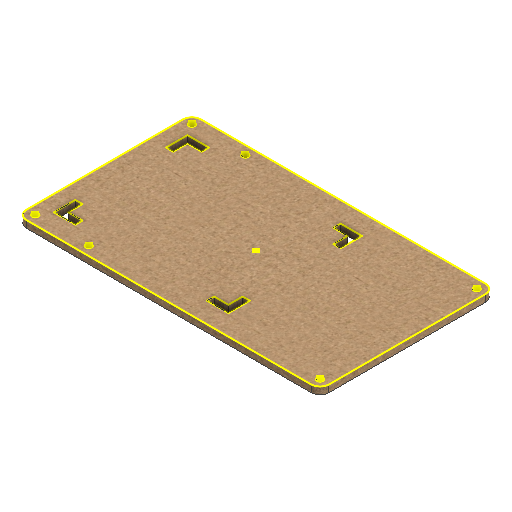
# Autodesk Inventor part: upper_plate
Saved by Autodesk Inventor 2025 (Build 290162000, 162)
## iProperties
Created: 2024-09-26
Part Number: upper_plate
Material: MDF Medium Density Fiberboard
Document SubType Name: Modeling
Designer: DANIEL
Density: 0.8 g/cm^3
Appearance: Cardboard - Corrugated
Checked By: FERNANDO
Engr Approved By: ANTONIO
Stock Number: 1
Author: DANIEL
Title: UPPER PLATE
Autodesk Inventor part; units mm, degrees
ref_plane "YZ Plane" through (0, 0, 0) normal (1, 0, 0) x (0, 1, 0)
ref_plane "XZ Plane" through (0, 0, 0) normal (0, 1, 0) x (-1, 0, 0)
ref_plane "XY Plane" through (0, 0, 0) normal (0, 0, 1) x (1, 0, 0)
sketch "Sketch1" plane through (0, 0, 0) normal (0, 1, 0) x (-1, 0, 0)
  line L0 (85, 49) -> (-85, 49)
  line L1 (-85, 49) -> (-85, -49)
  line L2 (-85, -49) -> (85, -49)
  line L3 (85, -49) -> (85, 49)
  line L4 (85, 49) -> (-85, -49) construction
  line L5 (-85, 49) -> (85, -49) construction
  circle A0 centre (80, -44) radius 1.7
  circle A1 centre (80, 44) radius 1.7
  circle A2 centre (-80, -44) radius 1.7
  circle A3 centre (-80, 44) radius 1.7
  circle A4 centre (50, -44) radius 1.7
  circle A5 centre (50, 44) radius 1.7
  point P0 (0, 0)
  dimension "d0" = 170
  dimension "d1" = 98
  dimension "d2" = 5
  dimension "d3" = 5
  dimension "d4" = 3.4
  dimension "d7" = 88
  dimension "d10" = 160
  dimension "d25" = 30
  constraints: 12 end point, 6 centre point, 4 coincident, 3 horizontal, 2 midpoint, 2 parallel, 1 perpendicular, 1 vertical, 13 other
  measures "d0" distance of L2.end L1.end
  measures "d1" distance of L1.end L0.end
  measures "d2" distance from line of L2 point (80, -44)
  measures "d3" distance from line of L3 point (80, -44)
  measures "d4" diameter of A0
  measures "d7" distance of A0.centre A1.centre
  measures "d10" distance of A0.centre A2.centre
  measures "d25" distance of A0.centre A4.centre
extrude "Extrusion1" add sketch "Sketch1" along normal blind 4
fillet "Fillet1" radius 5 4 edges at (85, 2, 49) (85, 2, -49) (-85, 2, 49) (-85, 2, -49)
sketch "Sketch2" plane through (0, 4, 0) normal (0, 1, 0) x (1, 0, 0)
  line L0 (-85, 44) -> (-85, -44) projected
  line L1 (-72, -33.5) -> (-62, -33.5)
  line L2 (-72, -37.5) -> (-72, -33.5)
  line L3 (-72, -23.5) -> (-72, -37.5)
  line L4 (18, 33.5) -> (10, 33.5)
  line L5 (10, 33.5) -> (10, 25.5)
  line L6 (10, 25.5) -> (18, 25.5)
  line L7 (18, 25.5) -> (18, 33.5)
  line L8 (10, 25.5) -> (22, 25.5)
  line L9 (22, 25.5) -> (22, 37.5)
  line L10 (22, 37.5) -> (10, 37.5)
  line L11 (10, 37.5) -> (10, 25.5)
  line L12 (-72, -33.5) -> (-64, -33.5)
  line L13 (-64, -33.5) -> (-64, -25.5)
  line L14 (-64, -25.5) -> (-72, -25.5)
  line L15 (-72, -25.5) -> (-72, -33.5)
  line L16 (-64, -25.5) -> (-76, -25.5)
  line L17 (-76, -25.5) -> (-76, -37.5)
  line L18 (-76, -37.5) -> (-64, -37.5)
  line L19 (-64, -37.5) -> (-64, -25.5)
  line L20 (-25.0039, 0) -> (-47.7766, 0)
  line L21 (-72, 33.5) -> (-62, 33.5)
  line L22 (-72, 37.5) -> (-72, 33.5)
  line L23 (-72, 23.5) -> (-72, 37.5)
  line L24 (18, -33.5) -> (10, -33.5)
  line L25 (10, -33.5) -> (10, -25.5)
  line L26 (10, -25.5) -> (18, -25.5)
  line L27 (18, -25.5) -> (18, -33.5)
  line L28 (10, -25.5) -> (22, -25.5)
  line L29 (22, -25.5) -> (22, -37.5)
  line L30 (22, -37.5) -> (10, -37.5)
  line L31 (10, -37.5) -> (10, -25.5)
  line L32 (-72, 33.5) -> (-64, 33.5)
  line L33 (-64, 33.5) -> (-64, 25.5)
  line L34 (-64, 25.5) -> (-72, 25.5)
  line L35 (-72, 25.5) -> (-72, 33.5)
  line L36 (-64, 25.5) -> (-76, 25.5)
  line L37 (-76, 25.5) -> (-76, 37.5)
  line L38 (-76, 37.5) -> (-64, 37.5)
  line L39 (-64, 37.5) -> (-64, 25.5)
  point P0 (0, 0)
  point P1 (10, 33.5)
  point P2 (18, 25.5)
  dimension "d30" = 13
  dimension "d31" = 33.5
  dimension "d36" = 67
  dimension "d37" = 90
  dimension "d38" = 8
  dimension "d39" = 8
  dimension "d40" = 12
  dimension "d41" = 12
  dimension "d44" = 8
  dimension "d45" = 8
  dimension "d46" = 12
  dimension "d47" = 12
  constraints: 78 end point, 17 symmetric about line, 8 parallel, 6 horizontal, 4 perpendicular
  measures "d30" distance from line of L0 L1.start
  measures "d31" vertical distance of point (0, 0) L1.start
  measures "d36" vertical distance of L1.start L4.start
  measures "d37" horizontal distance of L1.start L4.start
  measures "d38" distance of L6.end L5.end
  measures "d39" distance of L5.end L4.end
  measures "d40" distance of L10.end L9.end
  measures "d41" distance of L9.end L8.end
  measures "d44" distance of L14.end L13.end
  measures "d45" distance of L13.end L12.end
  measures "d46" distance of L18.end L17.end
  measures "d47" distance of L17.end L16.end
extrude "Extrusion2" cut sketch "Sketch2" against normal through all contours L1 L19 L18 L2 | L2 L18 L17 L16 L3 | L4 L11 L10 L9 L8 L7 | L22 L38 L39 L21 | L23 L36 L37 L38 L22 | L27 L28 L29 L30 L31 L24
sketch "Sketch3" plane through (0, 4, 0) normal (0, 1, 0) x (1, 0, 0)
  line L0 (-64, -33.5) -> (-64, -37.5) projected
  line L1 (-64, -37.5) -> (-76, -37.5) projected
  line L2 (-76, -37.5) -> (-76, -25.5) projected
  line L3 (-76, -25.5) -> (-72, -25.5) projected
  line L4 (-72, -25.5) -> (-72, -33.5) projected
  line L5 (-72, -33.5) -> (-64, -33.5) projected
  line L6 (18, -25.5) -> (22, -25.5) projected
  line L7 (22, -25.5) -> (22, -37.5) projected
  line L8 (22, -37.5) -> (10, -37.5) projected
  line L9 (10, -37.5) -> (10, -33.5) projected
  line L10 (10, -33.5) -> (18, -33.5) projected
  line L11 (18, -33.5) -> (18, -25.5) projected
  line L12 (18, 33.5) -> (10, 33.5) projected
  line L13 (10, 33.5) -> (10, 37.5) projected
  line L14 (10, 37.5) -> (22, 37.5) projected
  line L15 (22, 37.5) -> (22, 25.5) projected
  line L16 (22, 25.5) -> (18, 25.5) projected
  line L17 (18, 25.5) -> (18, 33.5) projected
  line L18 (-76, 25.5) -> (-76, 37.5) projected
  line L19 (-76, 37.5) -> (-64, 37.5) projected
  line L20 (-64, 37.5) -> (-64, 33.5) projected
  line L21 (-64, 33.5) -> (-72, 33.5) projected
  line L22 (-72, 33.5) -> (-72, 25.5) projected
  line L23 (-72, 25.5) -> (-76, 25.5) projected
  arc A0 (-80, 49) -> (-85, 44) centre (-80, 44) ccw projected
  line L24 (-85, 44) -> (-85, -44) projected
  arc A1 (-85, -44) -> (-80, -49) centre (-80, -44) ccw projected
  line L25 (-80, -49) -> (80, -49) projected
  arc A2 (80, -49) -> (85, -44) centre (80, -44) ccw projected
  line L26 (85, -44) -> (85, 44) projected
  arc A3 (85, 44) -> (80, 49) centre (80, 44) ccw projected
  line L27 (80, 49) -> (-80, 49) projected
  circle A4 centre (-80, 44) radius 1.7 projected
  circle A5 centre (-80, -44) radius 1.7 projected
  circle A6 centre (80, 44) radius 1.7 projected
  circle A7 centre (80, -44) radius 1.7 projected
  circle A8 centre (-50, 44) radius 1.7 projected
  circle A9 centre (-50, -44) radius 1.7 projected
  point P0 (0, 0)
equation "\"d39\" = d38"
equation "\"d41\" = d40"
equation "\"d44\" = d39"
equation "\"d45\" = d44"
equation "\"d46\" = d41"
equation "\"d47\" = d41"
body "Solid1"
